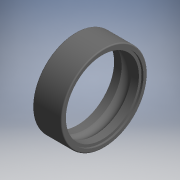
# Autodesk Inventor part: MR126ZZ Outer Ring
Saved by Autodesk Inventor 2017.3 (Build 213256000, 256)
## iProperties
Part Number: MR126ZZ Outer Ring
Material: Generic
Catalog Web Link: www.cadenas.de
Description: shielde_type_zz_zzs_OR-
Vendor: NSK_RB
Document SubType Name: Modeling
Designer: partserver
Manufacturer: NSK_RB
Mass: 0.110207 g
Surface Area: 3.45834 cm^2
Volume: 0.110207 cm^3
Density: 1 g/cm^3
Appearance: PSOLRGB-128-128-128
Category: PARTsolutions
Company: NSK_RB
Title: MR126ZZ Outer Ring
Author: Cadenas PARTsolutions
PSOL_IDENT_0: {$CADENAS_DATA\23d-libs\nsk_rb\roller_bearings\deep_groove_bb\exstra_small_miniatur_bb\metric_design
PSOL_IDENT_1: \shielded_type_zz_zzs_or.prj},193 {VTYP=3D},{NB=MR126ZZ Outer Ring},{LINA=MR126ZZ Outer Ring},{NN=sh
PSOL_IDENT_2: ielde_type_zz_zzs_OR},{DATE=16.07.2021 00:25:30},{GEOMDATE=04.01.2008 00:00:00},{VERSION=},{LINEID=5
PSOL_IDENT_3: 90},{WBVAR=},{WBNUMERIC=}  {NB=MR126ZZ Outer Ring},{LINA=MR126ZZ Outer Ring},{KT=DUMMY},{IDNR=},{STA
PSOL_IDENT_4: N=Standard},{ORDER=MR126ZZ},{SD=6.0},{X=6.0},{DI1=7.73},{DI2=7.20},{SDE1=10.19},{SDE2=10.90},{D=12},
PSOL_IDENT_5: {DD=12},{B=3.0},{B1=4.0},{R=0.20},{R1=0.15},{CR1=715},{COR1=292},{CR2=73},{COR2=30.0},{LG=43000},{LO=
PSOL_IDENT_6: 50000},{DA=0.0},{DB=7.2},{DA1=0.0},{DB1=10.9},{RA=0.00},{RB=0.15},{MASS=1.74},{SC=1}
NB: MR126ZZ Outer Ring
NN: shielde_type_zz_zzs_OR
NBSYN: $ORDER. Outer Ring
LINA: MR126ZZ Outer Ring
CATALOG: NSK Rolling Bearing
STAN: Standard
ORDER: MR126ZZ
SD: 6
X: 6
DI1: 7.73
DI2: 7.2
SDE1: 10.19
SDE2: 10.9
D: 12
DD: 12
B: 3
B1: 4
R: 0.2
R1: 0.15
CR1: 715
COR1: 292
CR2: 73
COR2: 30
LG: 43000
LO: 50000
DA: 0
DB: 7.2
DA1: 0
DB1: 10.9
RA: 0
RB: 0.15
MASS: 1.74
SC: 1
SUPPLIER: NSK_RB
ARTICLENO: MR126ZZ Outer Ring
BOMINFO: MR126ZZ Outer Ring
CREATOR: CADENAS GmbH
Autodesk Inventor part; units mm, degrees
sketch "Sketch_1" plane through (0, 0, 0) normal (0, 0, 1) x (1, 0, 0)
  line L0 (4, 0) -> (0, 0)
  line L1 (0, 5.45) -> (0.2656, 5.45)
  line L2 (0.2656, 5.45) -> (0.2656, 5.095)
  line L3 (0.2656, 5.095) -> (1.3247, 5.095)
  arc A0 (2.6753, 5.095) -> (1.3247, 5.095) centre (2, 4.5) ccw
  line L4 (2.6753, 5.095) -> (3.7344, 5.095)
  line L5 (3.7344, 5.095) -> (3.7344, 5.45)
  line L6 (3.7344, 5.45) -> (4, 5.45)
  line L7 (4, 5.45) -> (4, 5.85)
  arc A1 (4, 5.85) -> (3.85, 6) centre (3.85, 5.85) ccw
  line L8 (3.85, 6) -> (0.15, 6)
  arc A2 (0.15, 6) -> (0, 5.85) centre (0.15, 5.85) ccw
  line L9 (0, 5.85) -> (0, 5.45)
  constraints: 20 end point, 6 point on circle, 3 centre point
revolve "Revolution1" add sketch "Sketch_1" angle 360 about axis through (4, 0, 0) along (1, 0, 0)
ref_plane "ip_st_or_1_XY" through (0, 0, 0) normal (1, 0, 0) x (0, 0, -1)
ref_plane "ip_st_or_1_YZ" through (0, 0, 0) normal (0, 0, -1) x (0, 1, 0)
ref_plane "ip_st_or_1_ZX" through (0, 0, 0) normal (0, 1, 0) x (1, 0, 0)
ref_plane "ip_st_or_2_XY" through (3.7344, 0, 0) normal (-1, 0, 0) x (0, 0, -1)
ref_plane "ip_st_or_2_YZ" through (3.7344, 0, 0) normal (0, 0, -1) x (0, -1, 0)
ref_plane "ip_st_or_2_ZX" through (3.7344, 0, 0) normal (0, -1, 0) x (-1, 0, 0)
body "Solid1"
